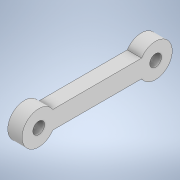
# Autodesk Inventor part: HexFlipperArmConnector
Saved by Autodesk Inventor 2020 (Build 240168000, 168)
## iProperties
Created: 2023-12-24
Part Number: HexFlipperArmConnector
Material: Generic
Document SubType Name: Modeling
Designer: smz3rm
Density: 1 g/cm^3
Appearance: Default
Author: smz3rm
Autodesk Inventor part; units mm, degrees
ref_plane "YZ Plane" through (0, 0, 0) normal (1, 0, 0) x (0, 1, 0)
ref_plane "XZ Plane" through (0, 0, 0) normal (0, 1, 0) x (-1, 0, 0)
ref_plane "XY Plane" through (0, 0, 0) normal (0, 0, 1) x (1, 0, 0)
sketch "Sketch1" plane through (0, 0, 0) normal (1, 0, 0) x (0, 1, 0)
  circle A0 centre (0, 0) radius 1.65
  circle A1 centre (0, -32.645) radius 1.65
  line L0 (0, -45.684) -> (0, 13.039) projected
  circle A2 centre (0, 0) radius 4.65
  circle A3 centre (0, -32.645) radius 4.65
  line L1 (2.5, -3.9208) -> (2.5, -28.7242)
  line L2 (-2.5, -3.9208) -> (-2.5, -28.7242)
  dimension "d0" = 3.3
  dimension "d1" = 32.645
  dimension "d2" = 3
  dimension "d3" = 3
  dimension "d4" = 5
  constraints: 4 centre point, 4 end point, 4 point on circle, 3 coincident, 2 parallel, 1 equal radius, 1 point on line, 1 vertical
  measures "d0" diameter of A0
  measures "d1" distance of A1.centre point (0, 0)
  measures "d2" radial gap between concentric circles of A2 A0
  measures "d3" radial gap between concentric circles of A3 A1
  measures "d4" distance between parallel lines of L2 L1
extrude "Extrusion1" add sketch "Sketch1" along normal blind 4 contours A0 L0 A2 | A0 L0 A2 | A2 L1 A3 L0 | L0 A3 L2 A2 | A3 L0 A1 | L0 A1 A3
equation "\"d1\" = FlipperArmConnectorLength"
equation "\"FlipperArmConnectorLength\" = 32.645"
body "Solid1"
